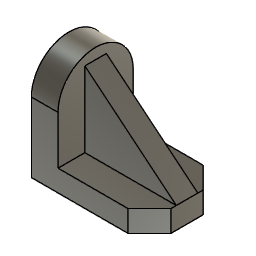
A1 (Autodesk Fusion 360 design; units mm, degrees)
Autodesk Fusion 360 part; units mm, degrees
note: some values were not read from the file. Chosen so that the rebuilt part matches the saved one: which pieces of a blend or face edit are solid.
sketch "Sketch1" plane through (0, 0, 0) normal (0, 0, 1) x (1, 0, 0)
  line L0 (-37.0773, 26.7781) -> (28.9227, 26.7781)
  line L1 (28.9227, 26.7781) -> (28.9227, -15.2219)
  line L2 (28.9227, -15.2219) -> (-37.0773, -15.2219)
  line L3 (-37.0773, -15.2219) -> (-37.0773, 26.7781)
  dimension "d1" = 66
  dimension "d2" = 42
  constraint horizontal L0
  constraint vertical L1
  constraint horizontal L2
  constraint vertical L3
  measures "d1" distance of L0.start L0.end
  measures "d2" distance of L0.start L2.end
extrude "Extrude1" add sketch "Sketch1" along normal blind 12
chamfer "Chamfer1" distance 12 angle 45 2 edges at (28.9227, -15.2219, 6) (28.9227, 26.7781, 6)
sketch "Sketch2" plane through (0, 0, 12) normal (0, 0, 1) x (-1, 0, 0)
  line L0 (-28.9227, -14.7781) -> (-16.9227, -26.7781)
  line L1 (-16.9227, -26.7781) -> (37.0773, -26.7781)
  line L2 (37.0773, -26.7781) -> (37.0773, 15.2219)
  line L3 (37.0773, 15.2219) -> (-16.9227, 15.2219)
  line L4 (-16.9227, 15.2219) -> (-28.9227, 3.2219)
  line L5 (-28.9227, 3.2219) -> (-28.9227, -14.7781)
  line L6 (37.0773, -26.7781) -> (22.184, -26.7781)
  line L7 (22.184, -26.7781) -> (22.184, 15.2219)
  line L8 (22.184, 15.2219) -> (37.0773, 15.2219)
  line L9 (37.0773, 15.2219) -> (37.0773, -26.7781)
  dimension "d6" = 14.8933
  constraint horizontal L6
  constraint vertical L7
  constraint horizontal L8
  constraint vertical L9
  constraint coincident L1.end L2.start
  measures "d6" distance of L1.end L6.end
extrude "Extrude2" add sketch "Sketch2" along normal blind 48 contours L1 L2 L3 L6 L7 L8 L9
fillet "Fillet1" radius 21 1 faces at (-32.1129, -1.2219, 60)
sketch "Sketch3" plane through (0, 0, 12) normal (0, 0, 1) x (-1, 0, 0)
  line L0 (22.184, -26.7781) -> (22.184, 15.2219)
  line L1 (22.184, 15.2219) -> (-16.9227, 15.2219)
  line L2 (-16.9227, 15.2219) -> (-28.9227, 3.2219)
  line L3 (-28.9227, 3.2219) -> (-28.9227, -14.7781)
  line L4 (-28.9227, -14.7781) -> (-16.9227, -26.7781)
  line L5 (-16.9227, -26.7781) -> (22.184, -26.7781)
  line L6 (-28.9227, -11.7781) -> (-28.9227, 0.2219)
  line L7 (-28.9227, 0.2219) -> (22.184, 0.2219)
  line L8 (-28.9227, -11.7781) -> (22.184, -11.7781)
  dimension "d12" = 12
  constraint coincident L3 L6.start
  constraint coincident L0 L7.end
  constraint perpendicular L0 L7
  constraint coincident L0 L8.end
  constraint perpendicular L0 L8
  measures "d12" distance of L6.start L6.end
extrude "Extrude3" add sketch "Sketch3" along normal blind 42 contours L0 L3 L6 L7 L8
chamfer "Chamfer2" distance 51.1 distance2 42 1 edges at (28.9227, 5.7781, 54) measured on face at (-5.1484, 7.7781, 54)
